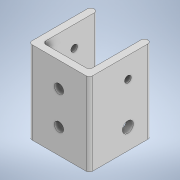
# Autodesk Inventor part: Long Robotics Mount V2
Saved by Autodesk Inventor 2020 (Build 240168000, 168)
## iProperties
Created: 2020-01-20
Part Number: Long Robotics Mount V2
Material: Generic
Document SubType Name: Modeling
Designer: maple
Density: 1 g/cm^3
Appearance: Default
Author: maple
Autodesk Inventor part; units mm, degrees
ref_plane "YZ Plane" through (0, 0, 0) normal (1, 0, 0) x (0, 1, 0)
ref_plane "XZ Plane" through (0, 0, 0) normal (0, 1, 0) x (-1, 0, 0)
ref_plane "XY Plane" through (0, 0, 0) normal (0, 0, 1) x (1, 0, 0)
sketch "Sketch1" plane through (0, 0, 0) normal (0, 1, 0) x (-1, 0, 0)
  line L0 (0, 0) -> (-21.59, 0)
  line L1 (-21.59, 0) -> (-21.59, -25.4)
  line L2 (-21.59, -25.4) -> (0, -25.4)
  line L3 (0, -25.4) -> (0, 0)
  line L4 (0, -25.4) -> (3.175, -25.4)
  line L5 (3.175, -25.4) -> (3.175, 3.175)
  line L6 (3.175, 3.175) -> (0, 3.175)
  line L7 (0, 3.175) -> (0, -25.4)
  line L8 (-21.59, -25.4) -> (-24.765, -25.4)
  line L9 (-24.765, -25.4) -> (-24.765, 3.175)
  line L10 (-24.765, 3.175) -> (-21.59, 3.175)
  line L11 (-21.59, 3.175) -> (-21.59, -25.4)
  line L12 (-21.59, 3.175) -> (0, 3.175)
  line L13 (0, 3.175) -> (0, 0)
  line L14 (0, 0) -> (-21.59, 0)
  line L15 (-21.59, 0) -> (-21.59, 3.175)
  dimension "d0" = 21.59
  dimension "d1" = 25.4
  dimension "d2" = 3.175
  dimension "d3" = 28.575
  dimension "d4" = 3.175
  constraints: 32 end point, 8 parallel, 4 horizontal, 4 perpendicular
  measures "d0" distance of L2.end L1.end
  measures "d1" distance of L1.end L0.end
  measures "d2" distance of L6.end L5.end
  measures "d3" distance of L5.end L4.end
  measures "d4" distance of L9.end L10.end
extrude "Extrusion1" add sketch "Sketch1" along normal blind 38.1 contours L7 L6 L5 L4 L3 | L0 L11 L12 L7 | L1 L8 L9 L10 L11
sketch "Sketch2" plane through (21.59, 0, 0) normal (0, 0, -1) x (-1, 0, 0)
  line L0 (24.765, 38.1) -> (-3.175, 38.1) projected
  line L1 (10.795, 38.1) -> (10.795, 26.67)
  line L2 (10.795, 38.1) -> (22.225, 38.1) construction
  line L3 (24.765, 0) -> (-3.175, 0) projected
  line L4 (10.795, 0) -> (10.795, 11.43)
  line L5 (10.795, 0) -> (22.225, 0) construction
  circle A0 centre (10.795, 26.67) radius 2.159
  circle A1 centre (10.795, 11.43) radius 2.159
  point P0 (21.59, 0)
  dimension "d7" = 11.43
  dimension "d8" = 90
  dimension "d9" = 11.43
  dimension "d10" = 90
  dimension "d11" = 4.318
  dimension "d12" = 4.318
  constraints: 8 end point, 2 centre point, 2 coincident, 2 horizontal, 2 midpoint, 2 perpendicular, 2 vertical
  measures "d7" distance of L1.start L1.end
  measures "d8" angle of L1 L2
  measures "d9" distance of L4.start L4.end
  measures "d10" angle of L5 L4
  measures "d11" diameter of A0
  measures "d12" diameter of A1
sketch "Sketch3" plane through (-3.175, 0, -25.4) normal (-1, 0, 0) x (0, 0, 1)
  line L0 (28.575, 38.1) -> (0, 38.1) projected
  line L1 (0, 38.1) -> (10.795, 38.1)
  line L2 (10.795, 38.1) -> (10.795, 28.575)
  line L3 (28.575, 0) -> (0, 0) projected
  line L4 (10.795, 0) -> (10.795, 9.525)
  line L5 (10.795, 0) -> (20.32, 0) construction
  circle A0 centre (10.795, 28.575) radius 1.524
  circle A1 centre (10.795, 9.525) radius 2.54
  point P0 (25.4, 0)
  dimension "d13" = 10.795
  dimension "d14" = 9.525
  dimension "d15" = 90
  dimension "d16" = 9.525
  dimension "d17" = 90
  dimension "d18" = 3.048
  dimension "d19" = 5.08
  constraints: 8 end point, 3 perpendicular, 2 centre point, 2 coincident, 2 point on line, 1 horizontal
  measures "d13" distance of L0.end L1.end
  measures "d14" distance of L1.end L2.end
  measures "d15" angle of L1 L2
  measures "d16" distance of L4.start L4.end
  measures "d17" angle of L5 L4
  measures "d18" diameter of A0
  measures "d19" diameter of A1
extrude "Extrusion2" cut sketch "Sketch2" against normal blind 38.1
extrude "Extrusion3" cut sketch "Sketch3" against normal blind 38.1
fillet "Fillet1" radius 1.524 7 edges at (-3.175, 19.05, 3.175) (0, 19.05, 0) (24.765, 19.05, -25.4) (21.59, 19.05, -25.4) (21.59, 19.05, 0) (0, 19.05, -25.4) (-3.175, 19.05, -25.4)
body "Solid1"
